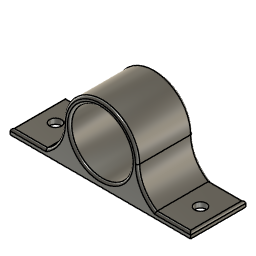
DrinkMixerV1PumpMount (Autodesk Fusion 360 design; units mm, degrees)
Autodesk Fusion 360 part; units mm, degrees
sketch "Sketch1" plane through (0, 0, 0) normal (0, 1, 0) x (1, 0, 0)
  circle A0 centre (0, 0) radius 14.5
  circle A1 centre (0, 0) radius 17.5
  line L0 (0, 17.5) -> (28.7095, 17.5) construction
  line L1 (17.5, 0) -> (17.5, 17.5) construction
  line L2 (17.5, 0) -> (17.5, 17.5)
  line L3 (0, 17.5) -> (17.5, 17.5)
  line L4 (17.5, 17.5) -> (42.5, 17.5)
  line L5 (42.5, 17.5) -> (42.5, 14.96)
  line L6 (42.5, 14.96) -> (17.5, 14.96)
  line L7 (17.5, 14.96) -> (17.5, 17.5)
  line L8 (17.5, 14.96) -> (18.9859, 14.96) construction
  line L9 (17.5, 14.96) -> (25.8, 14.96) construction
  arc A2 (25.8, 14.96) -> (17.5, 0) centre (35.132, 0) ccw
  line L10 (0, -17.5) -> (0, 17.5) construction
  line L11 (17.5, 0) -> (-17.5, 0) construction
  arc A3 (-17.5, 0) -> (-25.8, 14.96) centre (-35.132, 0) ccw
  line L12 (-17.5, 0) -> (-17.5, 17.5)
  line L13 (-17.5, 14.96) -> (-25.8, 14.96) construction
  line L14 (-42.5, 14.96) -> (-17.5, 14.96)
  line L15 (-42.5, 17.5) -> (-42.5, 14.96)
  line L16 (-17.5, 17.5) -> (-42.5, 17.5)
  line L17 (0, 17.5) -> (-17.5, 17.5)
  dimension "d5" = 29
  dimension "d6" = 35
  dimension "d7" = 25
  dimension "d8" = 2.54
  dimension "d9" = 8.3
  constraint coincident A0.centre A1.centre
  constraint coincident A1 L0.start
  constraint tangent A1 L0
  constraint horizontal L0
  constraint coincident A1 L1.start
  constraint coincident L0 L1.end
  constraint tangent A1 L1
  constraint perpendicular L0 L1
  constraint horizontal L4
  constraint vertical L5
  constraint horizontal L6
  constraint vertical L7
  constraint coincident L6 L8.end
  constraint perpendicular L2 L8
  constraint perpendicular L2 L9
  constraint tangent A1 A2
  constraint coincident A1 L10.start
  constraint perpendicular L3 L10
  constraint coincident A1 L11.end
  constraint perpendicular L1 L11
  constraint symmetric L0.start L10 L3.start
  constraint symmetric L1.start L10 L11.end
  constraint symmetric L1.end L10 L12.end
  constraint symmetric L4.end L10 L15.start
  constraint symmetric L5.end L10 L14.start
  constraint symmetric L6.end L10 L13.start
  constraint symmetric L9.end L10 A3.end
  constraint symmetric A2 L10 A3
  measures "d5" diameter of A0
  measures "d6" diameter of A1
  measures "d7" distance of L1.end L4.end
  measures "d8" distance of L1.end L6.end
  measures "d9" distance of L6.end L9.end
extrude "Extrude1" add sketch "Sketch1" along normal blind 26
sketch "Sketch3" plane through (0, 0, -14.96) normal (0, 0, 1) x (-1, 0, 0)
  line L0 (-25.8, 0) -> (-42.5, 0)
  line L1 (-42.5, 0) -> (-42.5, -26)
  line L2 (-42.5, -26) -> (-25.8, -26)
  line L3 (-25.8, -26) -> (-25.8, 0)
  line L4 (-25.8, -26) -> (-42.5, 0) construction
  line L5 (-42.5, -26) -> (-25.8, 0) construction
  circle A0 centre (-34.15, -13) radius 2.75
  dimension "d16" = 5.5
  constraint coincident L2.end L3.start
  constraint coincident L0.end L1.start
  constraint coincident L1.end L2.start
  constraint coincident L0.start L3.end
  constraint midpoint L4 A0.centre
  measures "d16" diameter of A0
extrude "Extrude2" cut sketch "Sketch3" against normal up to surface (2.54 mm away) contours A0
mirror "Mirror1" about plane through (0, 0, 0) normal (1, 0, 0) of "Extrude2"
fillet "Fillet3" radius 1 13 edges at (-34.15, 0, -14.96) (-42.5, 13, -14.96) (-34.15, 26, -14.96) (-19.714, 0, -8.5541) (0, 0, 17.5) (19.714, 0, -8.5541) (-13.5187, 0, -5.2434) (34.15, 26, -14.96) (-19.714, 26, -8.5541) (0, 26, 17.5) (19.714, 26, -8.5541) (34.15, 0, -14.96) (42.5, 13, -14.96)
equation "InnerDiameter = 29 mm"
equation "OuterDiameter = 35 mm"
equation "Width = 26 mm"
equation "ScrewDiameter = 5.5 mm"
equation "d5 = InnerDiameter"
equation "d6 = OuterDiameter"
equation "d10 = Width"
equation "d16 = ScrewDiameter"
